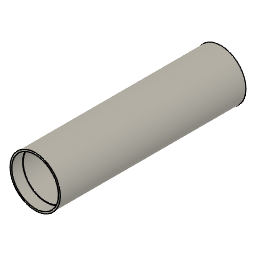
cad_native (Autodesk Fusion 360 archive; units mm, degrees)
design "Thermal Paste"
Autodesk Fusion 360 part; units mm, degrees
(part 1 of 3)
sketch "motor_base_geometry" plane through (0, 0, 0) normal (0, 1, 0) x (1, 0, 0)
  line L0 (0, 500) -> (0, 520)
  line L1 (5, -180) -> (5, -200)
  line L2 (0, 360) -> (0, 380)
  line L3 (5, -120) -> (5, -140)
  line L4 (0, 520) -> (0, 624)
  line L5 (0, 100) -> (0, 120)
  line L6 (0, 60) -> (0, 80)
  line L7 (6, -520) -> (6, 520)
  line L8 (0, 420) -> (0, 440)
  line L9 (5, 520) -> (5, 500)
  line L10 (0, -400) -> (0, -380)
  line L11 (5, -100) -> (5, -120)
  line L12 (5, -80) -> (5, -100)
  line L13 (0, -440) -> (0, -420)
  line L14 (0, 460) -> (0, 480)
  line L15 (0, -180) -> (0, -160)
  line L16 (0, -480) -> (0, -460)
  line L17 (0, -160) -> (0, -140)
  line L18 (5, -420) -> (5, -440)
  line L19 (5, -320) -> (5, -340)
  line L20 (5, -500) -> (0, -500)
  line L21 (0, -624) -> (0, -520)
  line L22 (5, -40) -> (5, -60)
  line L23 (0, 40) -> (0, 60)
  line L24 (5, -340) -> (5, -360)
  line L25 (5, 300) -> (5, 280)
  line L26 (0, 0) -> (0, 20)
  line L27 (0, 380) -> (0, 400)
  line L28 (5, 340) -> (5, 320)
  line L29 (5, -520) -> (6, -520)
  line L30 (5, 440) -> (5, 420)
  line L31 (0, 340) -> (0, 360)
  line L32 (5, -260) -> (5, -280)
  line L33 (0, 480) -> (0, 500)
  line L34 (5, 480) -> (5, 460)
  line L35 (5, 460) -> (5, 440)
  line L36 (0, -300) -> (0, -280)
  line L37 (0, -120) -> (0, -100)
  line L38 (5, 400) -> (5, 380)
  line L39 (0, 320) -> (0, 340)
  line L40 (5, 80) -> (5, 60)
  line L41 (0, 280) -> (0, 300)
  line L42 (26.7, 624) -> (26.7, -624)
  line L43 (0, -40) -> (0, -20)
  line L44 (0, -80) -> (0, -60)
  line L45 (5, 0) -> (5, -20)
  line L46 (0, 624) -> (26.7, 624)
  line L47 (5, 100) -> (5, 80)
  line L48 (0, 200) -> (0, 220)
  line L49 (5, -60) -> (5, -80)
  line L50 (0, 220) -> (0, 240)
  line L51 (5, 40) -> (5, 20)
  line L52 (0, -260) -> (0, -240)
  line L53 (0, 160) -> (0, 180)
  line L54 (5, 260) -> (5, 240)
  line L55 (0, 240) -> (0, 260)
  line L56 (0, 20) -> (0, 40)
  line L57 (0, 140) -> (0, 160)
  line L58 (0, 400) -> (0, 420)
  line L59 (0, 180) -> (0, 200)
  line L60 (0, -20) -> (0, 0)
  line L61 (0, -100) -> (0, -80)
  line L62 (5, 320) -> (5, 300)
  line L63 (5, 420) -> (5, 400)
  line L64 (5, 200) -> (5, 180)
  line L65 (5, -160) -> (5, -180)
  line L66 (0, -240) -> (0, -220)
  line L67 (0, -520) -> (5, -520)
  line L68 (6, 520) -> (5, 520)
  line L69 (0, -460) -> (0, -440)
  line L70 (5, -400) -> (5, -420)
  line L71 (5, -300) -> (5, -320)
  line L72 (5, 120) -> (5, 100)
  line L73 (5, 360) -> (5, 340)
  line L74 (5, 380) -> (5, 360)
  line L75 (5, 20) -> (5, 0)
  line L76 (5, -20) -> (5, -40)
  line L77 (0, -320) -> (0, -300)
  line L78 (0, -420) -> (0, -400)
  line L79 (5, -380) -> (5, -400)
  line L80 (5, -360) -> (5, -380)
  line L81 (5, -480) -> (5, -500)
  line L82 (5, -140) -> (5, -160)
  line L83 (0, -380) -> (0, -360)
  line L84 (0, -340) -> (0, -320)
  line L85 (5, 160) -> (5, 140)
  line L86 (0, -360) -> (0, -340)
  line L87 (5, 220) -> (5, 200)
  line L88 (5, -220) -> (5, -240)
  line L89 (5, 280) -> (5, 260)
  line L90 (0, -280) -> (0, -260)
  line L91 (5, 180) -> (5, 160)
  line L92 (5, 60) -> (5, 40)
  line L93 (5, -440) -> (5, -460)
  line L94 (5, 140) -> (5, 120)
  line L95 (5, -200) -> (5, -220)
  line L96 (5, 240) -> (5, 220)
  line L97 (5, 500) -> (5, 480)
  line L98 (5, -460) -> (5, -480)
  line L99 (0, -140) -> (0, -120)
  line L100 (0, -500) -> (0, -480)
  line L101 (5, -280) -> (5, -300)
  line L102 (0, -220) -> (0, -200)
  line L103 (5, -240) -> (5, -260)
  line L104 (0, 440) -> (0, 460)
  line L105 (26.7, -624) -> (0, -624)
  line L106 (0, 260) -> (0, 280)
  line L107 (0, -200) -> (0, -180)
  line L108 (0, 80) -> (0, 100)
  line L109 (0, 300) -> (0, 320)
  line L110 (0, 120) -> (0, 140)
  line L111 (0, -60) -> (0, -40)
  line L112 (10.5, -25.1667) -> (10.5, -30)
  line L113 (7.5, -25.1667) -> (10.5, -25.1667)
  line L114 (7.5, -30) -> (7.5, -25.1667)
  line L115 (10.5, -30) -> (7.5, -30)
  line L116 (7.5, -23.1667) -> (7.5, -18.3333)
  line L117 (7.5, -18.3333) -> (10.5, -18.3333)
  line L118 (10.5, -23.1667) -> (7.5, -23.1667)
  line L119 (10.5, -18.3333) -> (10.5, -23.1667)
  line L120 (10.5, -16.3333) -> (7.5, -16.3333)
  line L121 (7.5, -11.5) -> (10.5, -11.5)
  line L122 (10.5, -11.5) -> (10.5, -16.3333)
  line L123 (7.5, -16.3333) -> (7.5, -11.5)
  line L124 (10.5, -4.6667) -> (10.5, -9.5)
  line L125 (7.5, -9.5) -> (7.5, -4.6667)
  line L126 (7.5, -4.6667) -> (10.5, -4.6667)
  line L127 (10.5, -9.5) -> (7.5, -9.5)
  line L128 (10.5, -2.6667) -> (7.5, -2.6667)
  line L129 (10.5, 2.1667) -> (10.5, -2.6667)
  line L130 (7.5, 2.1667) -> (10.5, 2.1667)
  line L131 (7.5, -2.6667) -> (7.5, 2.1667)
  line L132 (7.5, 4.1667) -> (7.5, 9)
  line L133 (7.5, 9) -> (10.5, 9)
  line L134 (10.5, 9) -> (10.5, 4.1667)
  line L135 (10.5, 4.1667) -> (7.5, 4.1667)
  line L136 (10.5, 15.8333) -> (10.5, 11)
  line L137 (7.5, 15.8333) -> (10.5, 15.8333)
  line L138 (7.5, 11) -> (7.5, 15.8333)
  line L139 (10.5, 11) -> (7.5, 11)
  line L140 (10.5, 17.8333) -> (7.5, 17.8333)
  line L141 (7.5, 22.6667) -> (10.5, 22.6667)
  line L142 (10.5, 22.6667) -> (10.5, 17.8333)
  line L143 (7.5, 17.8333) -> (7.5, 22.6667)
  line L144 (10.5, 29.5) -> (10.5, 24.6667)
  line L145 (7.5, 29.5) -> (10.5, 29.5)
  line L146 (10.5, 24.6667) -> (7.5, 24.6667)
  line L147 (7.5, 24.6667) -> (7.5, 29.5)
  line L148 (10.5, 36.3333) -> (10.5, 31.5)
  line L149 (7.5, 31.5) -> (7.5, 36.3333)
  line L150 (7.5, 36.3333) -> (10.5, 36.3333)
  line L151 (10.5, 31.5) -> (7.5, 31.5)
  line L152 (7.5, 38.3333) -> (7.5, 43.1667)
  line L153 (7.5, 43.1667) -> (10.5, 43.1667)
  line L154 (10.5, 43.1667) -> (10.5, 38.3333)
  line L155 (10.5, 38.3333) -> (7.5, 38.3333)
  line L156 (10.5, 45.1667) -> (7.5, 45.1667)
  line L157 (7.5, 45.1667) -> (7.5, 50)
  line L158 (10.5, 50) -> (10.5, 45.1667)
  line L159 (7.5, 50) -> (10.5, 50)
  line L160 (10.5, 45.1667) -> (10.5, 43.1667)
  line L161 (10.5, 38.3333) -> (10.5, 36.3333)
  line L162 (10.5, 31.5) -> (10.5, 29.5)
  line L163 (10.5, 24.6667) -> (10.5, 22.6667)
  line L164 (10.5, 17.8333) -> (10.5, 15.8333)
  line L165 (10.5, 4.1667) -> (10.5, 2.1667)
  line L166 (10.5, -2.6667) -> (10.5, -4.6667)
  line L167 (10.5, -9.5) -> (10.5, -11.5)
  line L168 (10.5, -16.3333) -> (10.5, -18.3333)
  line L169 (10.5, -23.1667) -> (10.5, -25.1667)
  line L170 (17.8, -19.25) -> (17.8, -18.75)
  line L171 (6.5, -38) -> (17.8, -38)
  line L172 (9, -35) -> (6.5, -35)
  line L173 (17.8, -33.25) -> (17.8, -32.75)
  line L174 (12.3, -32.75) -> (12.3, -31.25)
  line L175 (17.8, -29.25) -> (17.8, -28.75)
  line L176 (12.3, -28.75) -> (12.3, -27.25)
  line L177 (17.8, -26.75) -> (12.3, -26.75)
  line L178 (12.3, -30.75) -> (12.3, -29.25)
  line L179 (12.3, -14.75) -> (12.3, -13.25)
  line L180 (12.3, -12.75) -> (12.3, -11.25)
  line L181 (17.8, -12.75) -> (12.3, -12.75)
  line L182 (12.3, -7.25) -> (17.8, -7.25)
  line L183 (17.8, -32.75) -> (12.3, -32.75)
  line L184 (17.8, -20.75) -> (12.3, -20.75)
  line L185 (17.8, -21.25) -> (17.8, -20.75)
  line L186 (12.3, -15.25) -> (17.8, -15.25)
  line L187 (10.7, -35) -> (9, -35)
  line L188 (17.8, -10.75) -> (12.3, -10.75)
  line L189 (17.8, -11.25) -> (17.8, -10.75)
  line L190 (12.3, -11.25) -> (17.8, -11.25)
  line L191 (17.8, -25.25) -> (17.8, -24.75)
  line L192 (17.8, 6.75) -> (17.8, 7.25)
  line L193 (17.8, -23.25) -> (17.8, -22.75)
  line L194 (12.3, 1.25) -> (12.3, 2.75)
  line L195 (12.3, -13.25) -> (17.8, -13.25)
  line L196 (17.8, -28.75) -> (12.3, -28.75)
  line L197 (12.3, -29.25) -> (17.8, -29.25)
  line L198 (11.5, -35) -> (10.7, -35)
  line L199 (17.8, 5.25) -> (12.3, 5.25)
  line L200 (12.3, -27.25) -> (17.8, -27.25)
  line L201 (12.3, 6.75) -> (17.8, 6.75)
  line L202 (12.3, 12.75) -> (17.8, 12.75)
  line L203 (17.8, 18.75) -> (17.8, 19.25)
  line L204 (12.3, -17.25) -> (17.8, -17.25)
  line L205 (12.3, -23.25) -> (17.8, -23.25)
  line L206 (12.3, -16.75) -> (12.3, -15.25)
  line L207 (11.5, -30) -> (11.5, -35)
  line L208 (12.3, -18.75) -> (12.3, -17.25)
  line L209 (17.8, -13.25) -> (17.8, -12.75)
  line L210 (17.8, -31.25) -> (17.8, -30.75)
  line L211 (17.8, -16.75) -> (12.3, -16.75)
  line L212 (17.8, -14.75) -> (12.3, -14.75)
  line L213 (6.5, -35) -> (6.5, -38)
  line L214 (17.8, -15.25) -> (17.8, -14.75)
  line L215 (17.8, 8.75) -> (17.8, 9.25)
  line L216 (12.3, 9.25) -> (12.3, 10.75)
  line L217 (12.3, 42.75) -> (17.8, 42.75)
  line L218 (12.3, 40.75) -> (17.8, 40.75)
  line L219 (12.3, 37.25) -> (12.3, 38.75)
  line L220 (12.3, 35.25) -> (12.3, 36.75)
  line L221 (12.3, 8.75) -> (17.8, 8.75)
  line L222 (12.3, 30.75) -> (17.8, 30.75)
  line L223 (17.8, 49.25) -> (12.3, 49.25)
  line L224 (17.8, 38.75) -> (17.8, 39.25)
  line L225 (17.8, 35.25) -> (12.3, 35.25)
  line L226 (17.8, 39.25) -> (12.3, 39.25)
  line L227 (12.3, -0.75) -> (12.3, 0.75)
  line L228 (12.3, 34.75) -> (17.8, 34.75)
  line L229 (17.8, 50.75) -> (17.8, 51.25)
  line L230 (11.5, 51.25) -> (11.5, 50)
  line L231 (12.3, 43.25) -> (12.3, 44.75)
  line L232 (17.8, 3.25) -> (12.3, 3.25)
  line L233 (12.3, 21.25) -> (12.3, 22.75)
  line L234 (11.5, 50) -> (11.5, -30)
  line L235 (17.8, 17.25) -> (12.3, 17.25)
  line L236 (17.8, 46.75) -> (17.8, 47.25)
  line L237 (12.3, 47.25) -> (12.3, 48.75)
  line L238 (12.3, 24.75) -> (17.8, 24.75)
  line L239 (17.8, 36.75) -> (17.8, 37.25)
  line L240 (12.3, 23.25) -> (12.3, 24.75)
  line L241 (17.8, 40.75) -> (17.8, 41.25)
  line L242 (12.3, 44.75) -> (17.8, 44.75)
  line L243 (17.8, 48.75) -> (17.8, 49.25)
  line L244 (12.3, 41.25) -> (12.3, 42.75)
  line L245 (12.3, 18.75) -> (17.8, 18.75)
  line L246 (17.8, 45.25) -> (12.3, 45.25)
  line L247 (12.3, 45.25) -> (12.3, 46.75)
  line L248 (12.3, 20.75) -> (17.8, 20.75)
  line L249 (17.8, 14.75) -> (17.8, 15.25)
  line L250 (12.3, 39.25) -> (12.3, 40.75)
  line L251 (17.8, 9.25) -> (12.3, 9.25)
  line L252 (12.3, 15.25) -> (12.3, 16.75)
  line L253 (17.8, -24.75) -> (12.3, -24.75)
  line L254 (17.8, -9.25) -> (17.8, -8.75)
  line L255 (17.8, 44.75) -> (17.8, 45.25)
  line L256 (12.3, 13.25) -> (12.3, 14.75)
  line L257 (12.3, -19.25) -> (17.8, -19.25)
  line L258 (17.8, 41.25) -> (12.3, 41.25)
  line L259 (17.8, -0.75) -> (12.3, -0.75)
  line L260 (17.8, 42.75) -> (17.8, 43.25)
  line L261 (12.3, -31.25) -> (17.8, -31.25)
  line L262 (17.8, -18.75) -> (12.3, -18.75)
  line L263 (12.3, -25.25) -> (17.8, -25.25)
  line L264 (12.3, -9.25) -> (17.8, -9.25)
  line L265 (12.3, -24.75) -> (12.3, -23.25)
  line L266 (12.3, -20.75) -> (12.3, -19.25)
  line L267 (12.3, -22.75) -> (12.3, -21.25)
  line L268 (17.8, -22.75) -> (12.3, -22.75)
  line L269 (17.8, 33.25) -> (12.3, 33.25)
  line L270 (17.8, -27.25) -> (17.8, -26.75)
  line L271 (12.3, 49.25) -> (12.3, 50.75)
  line L272 (17.8, -8.75) -> (12.3, -8.75)
  line L273 (12.3, 50.75) -> (17.8, 50.75)
  line L274 (17.8, -17.25) -> (17.8, -16.75)
  line L275 (12.3, 4.75) -> (17.8, 4.75)
  line L276 (12.3, -21.25) -> (17.8, -21.25)
  line L277 (17.8, -38) -> (17.8, -33.25)
  line L278 (17.8, 47.25) -> (12.3, 47.25)
  line L279 (12.3, -10.75) -> (12.3, -9.25)
  line L280 (17.8, -30.75) -> (12.3, -30.75)
  line L281 (12.3, -26.75) -> (12.3, -25.25)
  line L282 (12.3, -8.75) -> (12.3, -7.25)
  line L283 (17.8, -7.25) -> (17.8, -6.75)
  line L284 (17.8, -1.25) -> (17.8, -0.75)
  line L285 (17.8, 51.4522) -> (11.5, 51.4522)
  line L286 (12.3, 33.25) -> (12.3, 34.75)
  line L287 (12.3, 48.75) -> (17.8, 48.75)
  line L288 (17.8, 34.75) -> (17.8, 35.25)
  line L289 (12.3, 32.75) -> (17.8, 32.75)
  line L290 (17.8, 51.25) -> (17.8, 51.4522)
  line L291 (12.3, 36.75) -> (17.8, 36.75)
  line L292 (11.5, 51.4522) -> (11.5, 51.25)
  line L293 (17.8, 43.25) -> (12.3, 43.25)
  line L294 (17.8, 37.25) -> (12.3, 37.25)
  line L295 (12.3, 38.75) -> (17.8, 38.75)
  line L296 (12.3, 46.75) -> (17.8, 46.75)
  line L297 (17.8, 32.75) -> (17.8, 33.25)
  line L298 (12.3, 29.25) -> (12.3, 30.75)
  line L299 (17.8, 31.25) -> (12.3, 31.25)
  line L300 (12.3, 31.25) -> (12.3, 32.75)
  line L301 (17.8, -6.75) -> (12.3, -6.75)
  line L302 (12.3, 19.25) -> (12.3, 20.75)
  line L303 (17.8, 10.75) -> (17.8, 11.25)
  line L304 (17.8, 2.75) -> (17.8, 3.25)
  line L305 (17.8, 22.75) -> (17.8, 23.25)
  line L306 (12.3, -4.75) -> (12.3, -3.25)
  line L307 (17.8, 19.25) -> (12.3, 19.25)
  line L308 (17.8, -4.75) -> (12.3, -4.75)
  line L309 (12.3, 17.25) -> (12.3, 18.75)
  line L310 (17.8, 16.75) -> (17.8, 17.25)
  line L311 (17.8, 11.25) -> (12.3, 11.25)
  line L312 (17.8, 20.75) -> (17.8, 21.25)
  line L313 (12.3, 22.75) -> (17.8, 22.75)
  line L314 (17.8, 0.75) -> (17.8, 1.25)
  line L315 (12.3, 16.75) -> (17.8, 16.75)
  line L316 (17.8, 21.25) -> (12.3, 21.25)
  line L317 (12.3, 2.75) -> (17.8, 2.75)
  line L318 (12.3, -2.75) -> (12.3, -1.25)
  line L319 (12.3, 5.25) -> (12.3, 6.75)
  line L320 (17.8, 27.25) -> (12.3, 27.25)
  line L321 (12.3, -6.75) -> (12.3, -5.25)
  line L322 (12.3, -1.25) -> (17.8, -1.25)
  line L323 (17.8, -5.25) -> (17.8, -4.75)
  line L324 (17.8, 1.25) -> (12.3, 1.25)
  line L325 (17.8, 15.25) -> (12.3, 15.25)
  line L326 (17.8, 12.75) -> (17.8, 13.25)
  line L327 (12.3, -3.25) -> (17.8, -3.25)
  line L328 (12.3, 26.75) -> (17.8, 26.75)
  line L329 (17.8, 30.75) -> (17.8, 31.25)
  line L330 (17.8, -2.75) -> (12.3, -2.75)
  line L331 (12.3, 3.25) -> (12.3, 4.75)
  line L332 (12.3, 0.75) -> (17.8, 0.75)
  line L333 (12.3, 10.75) -> (17.8, 10.75)
  line L334 (12.3, 7.25) -> (12.3, 8.75)
  line L335 (17.8, 23.25) -> (12.3, 23.25)
  line L336 (17.8, 7.25) -> (12.3, 7.25)
  line L337 (17.8, 29.25) -> (12.3, 29.25)
  line L338 (12.3, 27.25) -> (12.3, 28.75)
  line L339 (17.8, -3.25) -> (17.8, -2.75)
  line L340 (17.8, 25.25) -> (12.3, 25.25)
  line L341 (17.8, 28.75) -> (17.8, 29.25)
  line L342 (17.8, 24.75) -> (17.8, 25.25)
  line L343 (12.3, 28.75) -> (17.8, 28.75)
  line L344 (17.8, 4.75) -> (17.8, 5.25)
  line L345 (17.8, 26.75) -> (17.8, 27.25)
  line L346 (12.3, 25.25) -> (12.3, 26.75)
  line L347 (17.8, 13.25) -> (12.3, 13.25)
  line L348 (12.3, -5.25) -> (17.8, -5.25)
  line L349 (12.3, 11.25) -> (12.3, 12.75)
  line L350 (12.3, 14.75) -> (17.8, 14.75)
  line L351 (6.5, -35) -> (6.5, 55)
  line L352 (0, -520) -> (0, -500)
  line L353 (5, -500) -> (5, -520)
  line L354 (0, -480) -> (5, -480)
  line L355 (0, -460) -> (5, -460)
  line L356 (0, -440) -> (5, -440)
  line L357 (0, -420) -> (5, -420)
  line L358 (0, -400) -> (5, -400)
  line L359 (0, -380) -> (5, -380)
  line L360 (0, -360) -> (5, -360)
  line L361 (0, -340) -> (5, -340)
  line L362 (0, -320) -> (5, -320)
  line L363 (0, -300) -> (5, -300)
  line L364 (0, -280) -> (5, -280)
  line L365 (0, -260) -> (5, -260)
  line L366 (0, -240) -> (5, -240)
  line L367 (0, -220) -> (5, -220)
  line L368 (0, -200) -> (5, -200)
  line L369 (0, -180) -> (5, -180)
  line L370 (0, -160) -> (5, -160)
  line L371 (0, -140) -> (5, -140)
  line L372 (0, -120) -> (5, -120)
  line L373 (0, -100) -> (5, -100)
  line L374 (0, -80) -> (5, -80)
  line L375 (0, -60) -> (5, -60)
  line L376 (0, -40) -> (5, -40)
  line L377 (0, -20) -> (5, -20)
  line L378 (0, 0) -> (5, 0)
  line L379 (0, 20) -> (5, 20)
  line L380 (0, 40) -> (5, 40)
  line L381 (0, 60) -> (5, 60)
  line L382 (0, 80) -> (5, 80)
  line L383 (0, 100) -> (5, 100)
  line L384 (0, 120) -> (5, 120)
  line L385 (0, 140) -> (5, 140)
  line L386 (0, 160) -> (5, 160)
  line L387 (0, 180) -> (5, 180)
  line L388 (0, 200) -> (5, 200)
  line L389 (0, 220) -> (5, 220)
  line L390 (0, 240) -> (5, 240)
  line L391 (0, 260) -> (5, 260)
  line L392 (0, 280) -> (5, 280)
  line L393 (0, 300) -> (5, 300)
  line L394 (0, 320) -> (5, 320)
  line L395 (0, 340) -> (5, 340)
  line L396 (0, 360) -> (5, 360)
  line L397 (0, 380) -> (5, 380)
  line L398 (0, 400) -> (5, 400)
  line L399 (0, 420) -> (5, 420)
  line L400 (0, 440) -> (5, 440)
  line L401 (0, 460) -> (5, 460)
  line L402 (0, 480) -> (5, 480)
  line L403 (0, 500) -> (5, 500)
  line L404 (0, 520) -> (5, 520)
  line L405 (17.8, -33.25) -> (12.3, -33.25)
  line L406 (12.3, -33.25) -> (12.3, -34.75)
  line L407 (10.5, 11) -> (10.5, 9)
  line L408 (12.3, -34.75) -> (12.3, -35)
  line L409 (12.3, -35) -> (11.5, -35)
  line L410 (9, -35) -> (9.1, -35)
  line L411 (12.3, -35) -> (12.4, -35)
  line L412 (12.4, -35) -> (12.4, -33.25)
  line L413 (10.5, 50) -> (11.4, 50)
  line L414 (11.4, 50) -> (11.4, 51.4522)
  line L415 (11.4, 51.4522) -> (11.5, 51.4522)
  line L416 (6.5, 55) -> (17.8, 55)
  line L417 (17.8, 55) -> (17.8, 51.4522)
  line L418 (10.5, -30) -> (10.7, -30)
  line L419 (10.7, -30) -> (10.7, -33)
  line L420 (10.7, -33) -> (10.7, -35)
  line L421 (11.5, 50) -> (11.4, 50)
  constraint perpendicular L414 L421
revolve "Revolve1" add sketch "motor_base_geometry" angle 360 about axis through (0, 0, 40) along (0, 0, -1) contours L112 L119 L122 L124 L129 L134 L136 L142 L144 L148 L154 L158 L160 L161 L162 L163 L164 L165 L166 L167 L168 L169 L198 L207 L234 L407 L413 L418 L419 L420 L421

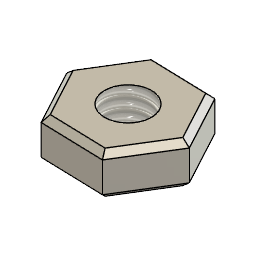
design "m2 nut"
Autodesk Fusion 360 part; units mm, degrees
sketch "Sketch1" plane through (0, 0, 0) normal (0, 1, 0) x (1, 0, 0)
  circle A0 centre (0, 0) radius 1
  line L0 (-1.0418, 1.9308) -> (-2.193, 0.0632)
  line L1 (-2.193, 0.0632) -> (-1.1513, -1.8676)
  line L2 (-1.1513, -1.8676) -> (1.0418, -1.9308)
  line L3 (1.0418, -1.9308) -> (2.193, -0.0632)
  line L4 (2.193, -0.0632) -> (1.1513, 1.8676)
  line L5 (1.1513, 1.8676) -> (-1.0418, 1.9308)
  dimension "d1" = 2
  dimension "d2" = 1.9
  constraint coincident A0.centre origin
  measures "d1" diameter of A0
  measures "d2" distance of A0.centre L5
extrude "Extrude1" add sketch "Sketch1" along normal blind 1.45
chamfer "Chamfer1" distance 0.2 angle 45 12 edges at (-1.6721, 1.45, 0.9022) (-0.0548, 1.45, 1.8992) (1.6174, 1.45, 0.997) (1.6721, 1.45, -0.9022) (0.0548, 1.45, -1.8992) (-1.6174, 1.45, -0.997) (-0.0548, 0, 1.8992) (-1.6721, 0, 0.9022) (1.6174, 0, 0.997) (1.6721, 0, -0.9022) (0.0548, 0, -1.8992) (-1.6174, 0, -0.997)
thread "Thread1" "ISO Metric profile 2.0 M2x0.4 M2x0.4 6H" major diameter 2.074 minor diameter 1.623 pitch 0.4 angle 60 resizes the face on face at (0.9988, 0.9667, 0.0498)
equation "d2 = ( 3.8 / 2 ) * 1 mm"

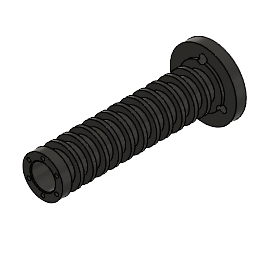
design "inner armature"
Autodesk Fusion 360 part; units mm, degrees
sketch "motor_base_geometry" plane through (0, 0, 0) normal (0, 1, 0) x (1, 0, 0)
  line L0 (0, -340) -> (0, -320)
  line L1 (0, 60) -> (0, 80)
  line L2 (5, 40) -> (5, 20)
  line L3 (5, -320) -> (5, -340)
  line L4 (5, 340) -> (5, 320)
  line L5 (6, -520) -> (6, 520)
  line L6 (0, -160) -> (0, -140)
  line L7 (5, 200) -> (5, 180)
  line L8 (5, -460) -> (5, -480)
  line L9 (0, -420) -> (0, -400)
  line L10 (5, 60) -> (5, 40)
  line L11 (5, 460) -> (5, 440)
  line L12 (5, -420) -> (5, -440)
  line L13 (5, 420) -> (5, 400)
  line L14 (5, 300) -> (5, 280)
  line L15 (5, -60) -> (5, -80)
  line L16 (5, 80) -> (5, 60)
  line L17 (5, 520) -> (5, 500)
  line L18 (5, 480) -> (5, 460)
  line L19 (5, 120) -> (5, 100)
  line L20 (0, -520) -> (5, -520)
  line L21 (0, -140) -> (0, -120)
  line L22 (0, -120) -> (0, -100)
  line L23 (0, 440) -> (0, 460)
  line L24 (0, 400) -> (0, 420)
  line L25 (5, 180) -> (5, 160)
  line L26 (5, -40) -> (5, -60)
  line L27 (0, -624) -> (0, -520)
  line L28 (5, 400) -> (5, 380)
  line L29 (5, 100) -> (5, 80)
  line L30 (5, 160) -> (5, 140)
  line L31 (5, 0) -> (5, -20)
  line L32 (5, -80) -> (5, -100)
  line L33 (5, 500) -> (5, 480)
  line L34 (5, 140) -> (5, 120)
  line L35 (5, 280) -> (5, 260)
  line L36 (0, 460) -> (0, 480)
  line L37 (5, 380) -> (5, 360)
  line L38 (0, -100) -> (0, -80)
  line L39 (5, 240) -> (5, 220)
  line L40 (5, -160) -> (5, -180)
  line L41 (6, 520) -> (5, 520)
  line L42 (5, 320) -> (5, 300)
  line L43 (0, 380) -> (0, 400)
  line L44 (5, 260) -> (5, 240)
  line L45 (0, 340) -> (0, 360)
  line L46 (0, -260) -> (0, -240)
  line L47 (0, 260) -> (0, 280)
  line L48 (0, -320) -> (0, -300)
  line L49 (5, -480) -> (5, -500)
  line L50 (5, -360) -> (5, -380)
  line L51 (26.7, -624) -> (0, -624)
  line L52 (0, 180) -> (0, 200)
  line L53 (0, 20) -> (0, 40)
  line L54 (0, 280) -> (0, 300)
  line L55 (0, -380) -> (0, -360)
  line L56 (0, 520) -> (0, 624)
  line L57 (5, 440) -> (5, 420)
  line L58 (0, 360) -> (0, 380)
  line L59 (0, 220) -> (0, 240)
  line L60 (0, 320) -> (0, 340)
  line L61 (0, -280) -> (0, -260)
  line L62 (5, -520) -> (6, -520)
  line L63 (5, -20) -> (5, -40)
  line L64 (0, -500) -> (0, -480)
  line L65 (0, 240) -> (0, 260)
  line L66 (5, -340) -> (5, -360)
  line L67 (0, 160) -> (0, 180)
  line L68 (0, -300) -> (0, -280)
  line L69 (5, 220) -> (5, 200)
  line L70 (0, -80) -> (0, -60)
  line L71 (0, 40) -> (0, 60)
  line L72 (0, -440) -> (0, -420)
  line L73 (5, -100) -> (5, -120)
  line L74 (0, -60) -> (0, -40)
  line L75 (5, -120) -> (5, -140)
  line L76 (5, -500) -> (0, -500)
  line L77 (0, -360) -> (0, -340)
  line L78 (5, -200) -> (5, -220)
  line L79 (5, 360) -> (5, 340)
  line L80 (5, -240) -> (5, -260)
  line L81 (5, 20) -> (5, 0)
  line L82 (5, -220) -> (5, -240)
  line L83 (0, -220) -> (0, -200)
  line L84 (5, -400) -> (5, -420)
  line L85 (0, -180) -> (0, -160)
  line L86 (5, -260) -> (5, -280)
  line L87 (5, -280) -> (5, -300)
  line L88 (5, -180) -> (5, -200)
  line L89 (0, -460) -> (0, -440)
  line L90 (5, -140) -> (5, -160)
  line L91 (5, -380) -> (5, -400)
  line L92 (5, -300) -> (5, -320)
  line L93 (0, -480) -> (0, -460)
  line L94 (0, -400) -> (0, -380)
  line L95 (5, -440) -> (5, -460)
  line L96 (0, -40) -> (0, -20)
  line L97 (0, -20) -> (0, 0)
  line L98 (0, 0) -> (0, 20)
  line L99 (0, 80) -> (0, 100)
  line L100 (0, 100) -> (0, 120)
  line L101 (0, 120) -> (0, 140)
  line L102 (0, 140) -> (0, 160)
  line L103 (0, 200) -> (0, 220)
  line L104 (0, 300) -> (0, 320)
  line L105 (0, -240) -> (0, -220)
  line L106 (0, -200) -> (0, -180)
  line L107 (0, 480) -> (0, 500)
  line L108 (0, 420) -> (0, 440)
  line L109 (0, 624) -> (26.7, 624)
  line L110 (26.7, 624) -> (26.7, -624)
  line L111 (0, 500) -> (0, 520)
  line L112 (10.5, -25.1667) -> (10.5, -30)
  line L113 (7.5, -25.1667) -> (10.5, -25.1667)
  line L114 (10.5, -30) -> (7.5, -30)
  line L115 (7.5, -30) -> (7.5, -25.1667)
  line L116 (10.5, -18.3333) -> (10.5, -23.1667)
  line L117 (10.5, -23.1667) -> (7.5, -23.1667)
  line L118 (7.5, -18.3333) -> (10.5, -18.3333)
  line L119 (7.5, -23.1667) -> (7.5, -18.3333)
  line L120 (7.5, -16.3333) -> (7.5, -11.5)
  line L121 (10.5, -16.3333) -> (7.5, -16.3333)
  line L122 (7.5, -11.5) -> (10.5, -11.5)
  line L123 (10.5, -11.5) -> (10.5, -16.3333)
  line L124 (7.5, -9.5) -> (7.5, -4.6667)
  line L125 (10.5, -4.6667) -> (10.5, -9.5)
  line L126 (10.5, -9.5) -> (7.5, -9.5)
  line L127 (7.5, -4.6667) -> (10.5, -4.6667)
  line L128 (7.5, -2.6667) -> (7.5, 2.1667)
  line L129 (7.5, 2.1667) -> (10.5, 2.1667)
  line L130 (10.5, -2.6667) -> (7.5, -2.6667)
  line L131 (10.5, 2.1667) -> (10.5, -2.6667)
  line L132 (10.5, 4.1667) -> (7.5, 4.1667)
  line L133 (7.5, 4.1667) -> (7.5, 9)
  line L134 (7.5, 9) -> (10.5, 9)
  line L135 (10.5, 9) -> (10.5, 4.1667)
  line L136 (10.5, 11) -> (7.5, 11)
  line L137 (10.5, 15.8333) -> (10.5, 11)
  line L138 (7.5, 15.8333) -> (10.5, 15.8333)
  line L139 (7.5, 11) -> (7.5, 15.8333)
  line L140 (10.5, 17.8333) -> (7.5, 17.8333)
  line L141 (7.5, 22.6667) -> (10.5, 22.6667)
  line L142 (10.5, 22.6667) -> (10.5, 17.8333)
  line L143 (7.5, 17.8333) -> (7.5, 22.6667)
  line L144 (7.5, 29.5) -> (10.5, 29.5)
  line L145 (10.5, 29.5) -> (10.5, 24.6667)
  line L146 (7.5, 24.6667) -> (7.5, 29.5)
  line L147 (10.5, 24.6667) -> (7.5, 24.6667)
  line L148 (10.5, 31.5) -> (7.5, 31.5)
  line L149 (7.5, 36.3333) -> (10.5, 36.3333)
  line L150 (7.5, 31.5) -> (7.5, 36.3333)
  line L151 (10.5, 36.3333) -> (10.5, 31.5)
  line L152 (7.5, 38.3333) -> (7.5, 43.1667)
  line L153 (10.5, 43.1667) -> (10.5, 38.3333)
  line L154 (10.5, 38.3333) -> (7.5, 38.3333)
  line L155 (7.5, 43.1667) -> (10.5, 43.1667)
  line L156 (10.5, 45.1667) -> (7.5, 45.1667)
  line L157 (7.5, 45.1667) -> (7.5, 50)
  line L158 (10.5, 50) -> (10.5, 45.1667)
  line L159 (7.5, 50) -> (10.5, 50)
  line L160 (10.5, 45.1667) -> (10.5, 43.1667)
  line L161 (10.5, 38.3333) -> (10.5, 36.3333)
  line L162 (10.5, 31.5) -> (10.5, 29.5)
  line L163 (10.5, 24.6667) -> (10.5, 22.6667)
  line L164 (10.5, 17.8333) -> (10.5, 15.8333)
  line L165 (10.5, 4.1667) -> (10.5, 2.1667)
  line L166 (10.5, -2.6667) -> (10.5, -4.6667)
  line L167 (10.5, -9.5) -> (10.5, -11.5)
  line L168 (10.5, -16.3333) -> (10.5, -18.3333)
  line L169 (10.5, -23.1667) -> (10.5, -25.1667)
  line L170 (17.8, 32.75) -> (17.8, 33.25)
  line L171 (17.8, -2.75) -> (12.3, -2.75)
  line L172 (17.8, 11.25) -> (12.3, 11.25)
  line L173 (17.8, 3.25) -> (12.3, 3.25)
  line L174 (12.3, 27.25) -> (12.3, 28.75)
  line L175 (12.3, 38.75) -> (17.8, 38.75)
  line L176 (12.3, 2.75) -> (17.8, 2.75)
  line L177 (11.5, 50) -> (11.5, -30)
  line L178 (17.8, 37.25) -> (12.3, 37.25)
  line L179 (12.3, 37.25) -> (12.3, 38.75)
  line L180 (17.8, 35.25) -> (12.3, 35.25)
  line L181 (17.8, -6.75) -> (12.3, -6.75)
  line L182 (12.3, 32.75) -> (17.8, 32.75)
  line L183 (17.8, 4.75) -> (17.8, 5.25)
  line L184 (12.3, -10.75) -> (12.3, -9.25)
  line L185 (17.8, 30.75) -> (17.8, 31.25)
  line L186 (17.8, 50.75) -> (17.8, 51.25)
  line L187 (12.3, 17.25) -> (12.3, 18.75)
  line L188 (11.5, 51.4522) -> (11.5, 51.25)
  line L189 (17.8, 42.75) -> (17.8, 43.25)
  line L190 (12.3, 49.25) -> (12.3, 50.75)
  line L191 (12.3, 42.75) -> (17.8, 42.75)
  line L192 (12.3, 29.25) -> (12.3, 30.75)
  line L193 (17.8, 25.25) -> (12.3, 25.25)
  line L194 (12.3, 21.25) -> (12.3, 22.75)
  line L195 (17.8, 43.25) -> (12.3, 43.25)
  line L196 (17.8, 47.25) -> (12.3, 47.25)
  line L197 (12.3, 24.75) -> (17.8, 24.75)
  line L198 (12.3, 45.25) -> (12.3, 46.75)
  line L199 (12.3, 41.25) -> (12.3, 42.75)
  line L200 (12.3, 44.75) -> (17.8, 44.75)
  line L201 (12.3, 47.25) -> (12.3, 48.75)
  line L202 (17.8, 38.75) -> (17.8, 39.25)
  line L203 (17.8, 27.25) -> (12.3, 27.25)
  line L204 (12.3, 31.25) -> (12.3, 32.75)
  line L205 (17.8, 23.25) -> (12.3, 23.25)
  line L206 (12.3, 43.25) -> (12.3, 44.75)
  line L207 (17.8, 45.25) -> (12.3, 45.25)
  line L208 (17.8, 40.75) -> (17.8, 41.25)
  line L209 (17.8, 44.75) -> (17.8, 45.25)
  line L210 (17.8, 12.75) -> (17.8, 13.25)
  line L211 (17.8, 0.75) -> (17.8, 1.25)
  line L212 (12.3, 13.25) -> (12.3, 14.75)
  line L213 (17.8, 6.75) -> (17.8, 7.25)
  line L214 (17.8, -8.75) -> (12.3, -8.75)
  line L215 (17.8, -1.25) -> (17.8, -0.75)
  line L216 (12.3, 8.75) -> (17.8, 8.75)
  line L217 (17.8, 16.75) -> (17.8, 17.25)
  line L218 (17.8, 19.25) -> (12.3, 19.25)
  line L219 (12.3, 18.75) -> (17.8, 18.75)
  line L220 (12.3, 20.75) -> (17.8, 20.75)
  line L221 (17.8, -3.25) -> (17.8, -2.75)
  line L222 (12.3, -3.25) -> (17.8, -3.25)
  line L223 (12.3, 10.75) -> (17.8, 10.75)
  line L224 (12.3, 11.25) -> (12.3, 12.75)
  line L225 (12.3, -4.75) -> (12.3, -3.25)
  line L226 (12.3, 0.75) -> (17.8, 0.75)
  line L227 (12.3, 15.25) -> (12.3, 16.75)
  line L228 (17.8, 21.25) -> (12.3, 21.25)
  line L229 (17.8, 8.75) -> (17.8, 9.25)
  line L230 (12.3, 1.25) -> (12.3, 2.75)
  line L231 (17.8, 9.25) -> (12.3, 9.25)
  line L232 (12.3, -7.25) -> (17.8, -7.25)
  line L233 (17.8, -4.75) -> (12.3, -4.75)
  line L234 (17.8, 5.25) -> (12.3, 5.25)
  line L235 (17.8, 18.75) -> (17.8, 19.25)
  line L236 (12.3, -6.75) -> (12.3, -5.25)
  line L237 (17.8, 13.25) -> (12.3, 13.25)
  line L238 (12.3, 14.75) -> (17.8, 14.75)
  line L239 (17.8, -0.75) -> (12.3, -0.75)
  line L240 (17.8, 15.25) -> (12.3, 15.25)
  line L241 (12.3, 6.75) -> (17.8, 6.75)
  line L242 (17.8, 2.75) -> (17.8, 3.25)
  line L243 (17.8, 14.75) -> (17.8, 15.25)
  line L244 (12.3, 12.75) -> (17.8, 12.75)
  line L245 (12.3, -2.75) -> (12.3, -1.25)
  line L246 (12.3, 19.25) -> (12.3, 20.75)
  line L247 (12.3, 4.75) -> (17.8, 4.75)
  line L248 (12.3, -0.75) -> (12.3, 0.75)
  line L249 (17.8, -7.25) -> (17.8, -6.75)
  line L250 (17.8, -5.25) -> (17.8, -4.75)
  line L251 (12.3, 7.25) -> (12.3, 8.75)
  line L252 (17.8, 1.25) -> (12.3, 1.25)
  line L253 (12.3, -9.25) -> (17.8, -9.25)
  line L254 (17.8, 39.25) -> (12.3, 39.25)
  line L255 (17.8, 31.25) -> (12.3, 31.25)
  line L256 (17.8, 20.75) -> (17.8, 21.25)
  line L257 (17.8, 46.75) -> (17.8, 47.25)
  line L258 (17.8, 10.75) -> (17.8, 11.25)
  line L259 (12.3, 5.25) -> (12.3, 6.75)
  line L260 (17.8, 49.25) -> (12.3, 49.25)
  line L261 (12.3, 16.75) -> (17.8, 16.75)
  line L262 (17.8, 17.25) -> (12.3, 17.25)
  line L263 (17.8, 7.25) -> (12.3, 7.25)
  line L264 (17.8, 28.75) -> (17.8, 29.25)
  line L265 (17.8, 34.75) -> (17.8, 35.25)
  line L266 (17.8, 22.75) -> (17.8, 23.25)
  line L267 (12.3, -5.25) -> (17.8, -5.25)
  line L268 (12.3, 9.25) -> (12.3, 10.75)
  line L269 (17.8, 51.25) -> (17.8, 51.4522)
  line L270 (12.3, 39.25) -> (12.3, 40.75)
  line L271 (12.3, 30.75) -> (17.8, 30.75)
  line L272 (12.3, 22.75) -> (17.8, 22.75)
  line L273 (12.3, -1.25) -> (17.8, -1.25)
  line L274 (11.5, 51.25) -> (11.5, 50)
  line L275 (17.8, 48.75) -> (17.8, 49.25)
  line L276 (12.3, 36.75) -> (17.8, 36.75)
  line L277 (12.3, 46.75) -> (17.8, 46.75)
  line L278 (17.8, 41.25) -> (12.3, 41.25)
  line L279 (17.8, 24.75) -> (17.8, 25.25)
  line L280 (17.8, -9.25) -> (17.8, -8.75)
  line L281 (12.3, 26.75) -> (17.8, 26.75)
  line L282 (17.8, 29.25) -> (12.3, 29.25)
  line L283 (17.8, 26.75) -> (17.8, 27.25)
  line L284 (12.3, 50.75) -> (17.8, 50.75)
  line L285 (12.3, 48.75) -> (17.8, 48.75)
  line L286 (12.3, 25.25) -> (12.3, 26.75)
  line L287 (12.3, 23.25) -> (12.3, 24.75)
  line L288 (12.3, 3.25) -> (12.3, 4.75)
  line L289 (12.3, 33.25) -> (12.3, 34.75)
  line L290 (12.3, 34.75) -> (17.8, 34.75)
  line L291 (17.8, -29.25) -> (17.8, -28.75)
  line L292 (17.8, -12.75) -> (12.3, -12.75)
  line L293 (11.5, -35) -> (10.7, -35)
  line L294 (12.3, 40.75) -> (17.8, 40.75)
  line L295 (6.5, -38) -> (17.8, -38)
  line L296 (12.3, -8.75) -> (12.3, -7.25)
  line L297 (12.3, 28.75) -> (17.8, 28.75)
  line L298 (12.3, -32.75) -> (12.3, -31.25)
  line L299 (17.8, 51.4522) -> (11.5, 51.4522)
  line L300 (17.8, -30.75) -> (12.3, -30.75)
  line L301 (12.3, -11.25) -> (17.8, -11.25)
  line L302 (17.8, -21.25) -> (17.8, -20.75)
  line L303 (17.8, -18.75) -> (12.3, -18.75)
  line L304 (12.3, -23.25) -> (17.8, -23.25)
  line L305 (12.3, 35.25) -> (12.3, 36.75)
  line L306 (12.3, -22.75) -> (12.3, -21.25)
  line L307 (17.8, -27.25) -> (17.8, -26.75)
  line L308 (17.8, 33.25) -> (12.3, 33.25)
  line L309 (17.8, -33.25) -> (17.8, -32.75)
  line L310 (6.5, -34.9518) -> (6.5, -38)
  line L311 (12.3, -15.25) -> (17.8, -15.25)
  line L312 (12.3, -17.25) -> (17.8, -17.25)
  line L313 (12.3, -25.25) -> (17.8, -25.25)
  line L314 (17.8, -15.25) -> (17.8, -14.75)
  line L315 (12.3, -30.75) -> (12.3, -29.25)
  line L316 (17.8, -38) -> (17.8, -33.25)
  line L317 (12.3, -28.75) -> (12.3, -27.25)
  line L318 (17.8, -24.75) -> (12.3, -24.75)
  line L319 (17.8, -32.75) -> (12.3, -32.75)
  line L320 (17.8, -10.75) -> (12.3, -10.75)
  line L321 (17.8, -26.75) -> (12.3, -26.75)
  line L322 (17.8, -25.25) -> (17.8, -24.75)
  line L323 (12.3, -26.75) -> (12.3, -25.25)
  line L324 (17.8, -17.25) -> (17.8, -16.75)
  line L325 (12.3, -13.25) -> (17.8, -13.25)
  line L326 (12.3, -19.25) -> (17.8, -19.25)
  line L327 (17.8, -13.25) -> (17.8, -12.75)
  line L328 (17.8, -14.75) -> (12.3, -14.75)
  line L329 (12.3, -24.75) -> (12.3, -23.25)
  line L330 (12.3, -14.75) -> (12.3, -13.25)
  line L331 (17.8, -19.25) -> (17.8, -18.75)
  line L332 (12.3, -31.25) -> (17.8, -31.25)
  line L333 (17.8, -20.75) -> (12.3, -20.75)
  line L334 (12.3, -27.25) -> (17.8, -27.25)
  line L335 (12.3, -18.75) -> (12.3, -17.25)
  line L336 (17.8, -28.75) -> (12.3, -28.75)
  line L337 (17.8, -31.25) -> (17.8, -30.75)
  line L338 (17.8, -11.25) -> (17.8, -10.75)
  line L339 (12.3, -29.25) -> (17.8, -29.25)
  line L340 (17.8, -16.75) -> (12.3, -16.75)
  line L341 (11.5, -30) -> (11.5, -35)
  line L342 (17.8, -23.25) -> (17.8, -22.75)
  line L343 (12.3, -12.75) -> (12.3, -11.25)
  line L344 (12.3, -20.75) -> (12.3, -19.25)
  line L345 (17.8, 36.75) -> (17.8, 37.25)
  line L346 (17.8, -22.75) -> (12.3, -22.75)
  line L347 (12.3, -21.25) -> (17.8, -21.25)
  line L348 (12.3, -16.75) -> (12.3, -15.25)
  line L349 (6.5, -34.9518) -> (6.5, 55)
  line L350 (0, -520) -> (0, -500)
  line L351 (5, -500) -> (5, -520)
  line L352 (0, -480) -> (5, -480)
  line L353 (0, -460) -> (5, -460)
  line L354 (0, -440) -> (5, -440)
  line L355 (0, -420) -> (5, -420)
  line L356 (0, -400) -> (5, -400)
  line L357 (0, -380) -> (5, -380)
  line L358 (0, -360) -> (5, -360)
  line L359 (0, -340) -> (5, -340)
  line L360 (0, -320) -> (5, -320)
  line L361 (0, -300) -> (5, -300)
  line L362 (0, -280) -> (5, -280)
  line L363 (0, -260) -> (5, -260)
  line L364 (0, -240) -> (5, -240)
  line L365 (0, -220) -> (5, -220)
  line L366 (0, -200) -> (5, -200)
  line L367 (0, -180) -> (5, -180)
  line L368 (0, -160) -> (5, -160)
  line L369 (0, -140) -> (5, -140)
  line L370 (0, -120) -> (5, -120)
  line L371 (0, -100) -> (5, -100)
  line L372 (0, -80) -> (5, -80)
  line L373 (0, -60) -> (5, -60)
  line L374 (0, -40) -> (5, -40)
  line L375 (0, -20) -> (5, -20)
  line L376 (0, 0) -> (5, 0)
  line L377 (0, 20) -> (5, 20)
  line L378 (0, 40) -> (5, 40)
  line L379 (0, 60) -> (5, 60)
  line L380 (0, 80) -> (5, 80)
  line L381 (0, 100) -> (5, 100)
  line L382 (0, 120) -> (5, 120)
  line L383 (0, 140) -> (5, 140)
  line L384 (0, 160) -> (5, 160)
  line L385 (0, 180) -> (5, 180)
  line L386 (0, 200) -> (5, 200)
  line L387 (0, 220) -> (5, 220)
  line L388 (0, 240) -> (5, 240)
  line L389 (0, 260) -> (5, 260)
  line L390 (0, 280) -> (5, 280)
  line L391 (0, 300) -> (5, 300)
  line L392 (0, 320) -> (5, 320)
  line L393 (0, 340) -> (5, 340)
  line L394 (0, 360) -> (5, 360)
  line L395 (0, 380) -> (5, 380)
  line L396 (0, 400) -> (5, 400)
  line L397 (0, 420) -> (5, 420)
  line L398 (0, 440) -> (5, 440)
  line L399 (0, 460) -> (5, 460)
  line L400 (0, 480) -> (5, 480)
  line L401 (0, 500) -> (5, 500)
  line L402 (0, 520) -> (5, 520)
  line L403 (17.8, -33.25) -> (12.3, -33.25)
  line L404 (12.3, -33.25) -> (12.3, -34.75)
  line L405 (10.5, 11) -> (10.5, 9)
  line L406 (12.3, -34.75) -> (12.3, -35)
  line L407 (12.3, -35) -> (11.5, -35)
  line L408 (12.3, -35) -> (12.4, -35)
  line L409 (12.4, -35) -> (12.4, -33.25)
  line L410 (10.5, 50) -> (11.4, 50)
  line L411 (11.4, 50) -> (11.4, 51.4522)
  line L412 (11.4, 51.4522) -> (11.5, 51.4522)
  line L413 (10.5, -30) -> (10.7, -30)
  line L414 (10.7, -30) -> (10.7, -33)
  line L415 (10.7, -33) -> (10.7, -35)
  line L416 (10.7, -35) -> (6.5, -35)
  line L417 (17.8, 51.4522) -> (17.8, 55)
  line L418 (17.8, 55) -> (6.5, 55)
  constraint coincident L310 L416.end
  constraint perpendicular L310 L416
  constraint perpendicular L299 L417
  constraint horizontal L418
revolve "Revolve1" add sketch "motor_base_geometry" angle 360 about axis through (0, 0, 40) along (0, 0, -1) contours L113 L114 L115 L117 L118 L119 L120 L121 L122 L124 L126 L127 L128 L129 L130 L132 L133 L134 L136 L138 L139 L140 L141 L143 L144 L146 L147 L148 L149 L150 L152 L154 L155 L156 L157 L159 L160 L161 L162 L163 L164 L165 L166 L167 L168 L169 L299 L310 L349 L405 L410 L411 L412 L413 L414 L415 L416 L417 L418
sketch "M2 Front mounting" plane through (0, 0, 35) normal (0, 0, 1) x (1, 0, 0)
  circle A0 centre (0, 0) radius 10.7
  circle A1 centre (0, 0) radius 6.5
  circle A2 centre (0, 0) radius 6.5 construction
  circle A3 centre (0, 0) radius 10.7 construction
  line L0 (0, 0) -> (0, 6.5) construction
  line L1 (0, 6.5) -> (0, 10.7) construction
  circle A4 centre (0, 8.6) radius 1
  circle A5 centre (-7.4478, 4.3) radius 1
  circle A6 centre (-7.4478, -4.3) radius 1
  circle A7 centre (0, -8.6) radius 1
  circle A8 centre (7.4478, -4.3) radius 1
  circle A9 centre (7.4478, 4.3) radius 1
  dimension "d2" = 2
  dimension "d16" = 360
  constraint coincident A0.centre A1.centre
  constraint coincident A2 L0.end
  constraint vertical L0
  constraint coincident A3 L1.end
  constraint parallel L0 L1
  constraint midpoint L1 A4.centre
  measures "d2" diameter of A4
extrude "Extrude1" cut sketch "M2 Front mounting" against normal blind 4 contours A4 | A5 | A6 | A7 | A8 | A9
extrude "Extrude2" add 1 faces at (13.9429, 1.2072, -55) along direction (0, 0, -1) blind 1.452
sketch "M3 Inserts Back mounting" plane through (0, 0, -56.452) normal (0, 0, -1) x (-1, 0, 0)
  circle A0 centre (0, 0) radius 6.5
  circle A1 centre (0, 0) radius 17.8
  line L0 (0, 0) -> (0, 6.5) construction
  line L1 (0, 6.5) -> (0, 17.8) construction
  circle A2 centre (0, 12.15) radius 2
  circle A3 centre (-10.5222, -6.075) radius 2
  circle A4 centre (10.5222, -6.075) radius 2
  dimension "d9" = 4
  dimension "d13" = 360
  constraint coincident A0.centre A1.centre
  constraint coincident A0 L0.end
  constraint vertical L0
  constraint coincident A1 L1.end
  constraint parallel L0 L1
  constraint midpoint L1 A2.centre
  measures "d9" diameter of A2
extrude "Extrude3" cut sketch "M3 Inserts Back mounting" against normal blind 7 contours A2 | A3 | A4
chamfer "Chamfer1" distance 0.4 angle 45 2 edges at (-6.0601, -2.3505, 35) (-6.0601, -2.3505, -56.452)
extrude "Extrude4" add 1 faces at (11.7971, -0.1479, -56.452) along direction (0, 0, -1) blind 0.298
named bodies: "main"

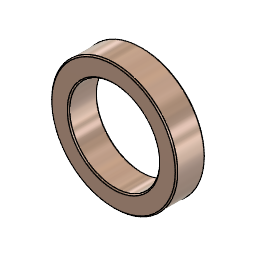
design "coil"
Autodesk Fusion 360 part; units mm, degrees